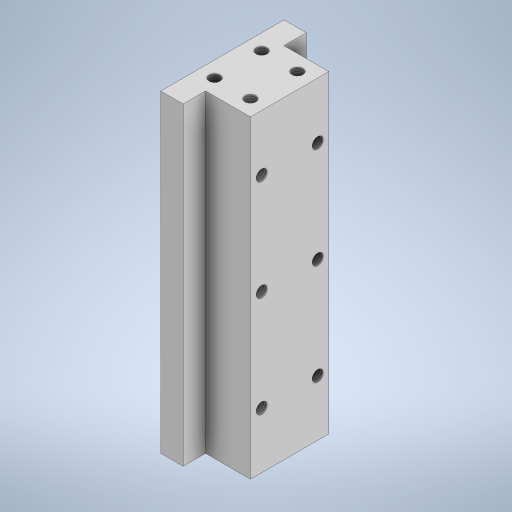
# Autodesk Inventor part: Fuhrung
Saved by Autodesk Inventor 2023 (Build 270158000, 158)
## iProperties
Created: 2023-05-10
Part Number: Fuhrung
Material: Generic
Document SubType Name: Modeling
Designer: dell
Density: 1 g/cm^3
Appearance: Default
Author: dell
Autodesk Inventor part; units mm, degrees
ref_plane "YZ Plane" through (0, 0, 0) normal (1, 0, 0) x (0, 1, 0)
ref_plane "XZ Plane" through (0, 0, 0) normal (0, 1, 0) x (-1, 0, 0)
ref_plane "XY Plane" through (0, 0, 0) normal (0, 0, 1) x (1, 0, 0)
sketch "Sketch1" plane through (0, 0, 0) normal (0, 1, 0) x (-1, 0, 0)
  line L0 (-10, 17.5) -> (10, 17.5)
  line L1 (10, 17.5) -> (10, -17.5)
  line L2 (10, -17.5) -> (-10, -17.5)
  line L3 (-10, -17.5) -> (-10, 17.5)
  line L4 (-10, 17.5) -> (10, -17.5) construction
  line L5 (10, 17.5) -> (-10, -17.5) construction
  point P0 (0, 0)
  dimension "d0" = 35
  dimension "d1" = 20
  constraints: 12 end point, 2 midpoint, 2 parallel, 1 horizontal, 1 perpendicular
  measures "d0" distance of L0.end L1.end
  measures "d1" distance of L1.end L2.end
extrude "Extrusion1" add sketch "Sketch1" along normal blind 140
sketch "Sketch2" plane through (0, 140, 0) normal (0, 1, 0) x (1, 0, 0)
  line L0 (-10, 27.5) -> (-10, -27.5)
  line L1 (-10, -27.5) -> (-20, -27.5)
  line L2 (-10, 27.5) -> (-20, 27.5)
  line L3 (-20, 27.5) -> (-20, -27.5)
  line L4 (-10, 17.5) -> (-10, -17.5) projected
  point P0 (0, 0)
  dimension "d4" = 55
  dimension "d5" = 0
  dimension "d6" = 10
  dimension "d7" = 27.5
  constraints: 8 end point, 2 horizontal, 2 vertical
  measures "d4" distance of L2.end L1.end
  measures "d5" distance between parallel lines of L0 L4
  measures "d6" distance between parallel lines of L0 L3
  measures "d7" distance from line of point (0, 0) L2
extrude "Extrusion2" add sketch "Sketch2" against normal blind 140
sketch "Sketch3" plane through (0, 140, 0) normal (0, 1, 0) x (1, 0, 0)
  line L0 (10, -17.5) -> (10, 17.5) projected
  point P0 (0, 0)
  point P1 (3, -10.5)
  dimension "d10" = 7
  dimension "d11" = 10.5
  measures "d10" distance from line of L0 point (3, -10.5)
  measures "d11" vertical distance of point (3, -10.5) point (0, 0)
hole "Hole1" at (3, 140, 10.5) direction (0, -1, 0) diameter 4.917 depth 20 tip angle 118 thread size "M6x1" class "6H" standard "ISO Metric profile"
pattern_linear "Rectangular Pattern1" count 2 spacing 16 along (-1, 0, 0) count 2 spacing 21 along (0, 0, -1) of "Hole1"
sketch "Sketch4" plane through (0, 0, 0) normal (0, -1, 0) x (1, 0, 0)
  line L0 (10, 17.5) -> (10, -17.5) projected
  point P0 (0, 0)
  point P1 (-13, -10.5)
  point P2 (-13, 10.5)
  point P3 (2, 0)
  dimension "d25" = 21
  dimension "d27" = 10.5
  dimension "d28" = 23
  dimension "d29" = 23
  dimension "d30" = 8
  dimension "d31" = 15
  measures "d25" distance of point (-13, -10.5) point (-13, 10.5)
  measures "d27" vertical distance of point (0, 0) point (-13, -10.5)
  measures "d28" distance from line of L0 point (-13, -10.5)
  measures "d29" distance from line of L0 point (-13, 10.5)
  measures "d30" distance from line of L0 point (2, 0)
  measures "d31" horizontal distance of point (-13, 10.5) point (2, 0)
hole "Hole2" at (-13, 0, -10.5) at (-13, 0, 10.5) at (2, 0, 0) direction (0, 1, 0) diameter 6.647 depth 20 tip angle 118 thread size "M8x1.25" class "6H" standard "ISO Metric profile"
sketch "Sketch5" plane through (10, 0, 17.5) normal (1, 0, 0) x (0, 0, -1)
  line L0 (0, 0) -> (35, 0) projected
  point P0 (17.5, 0)
  point P1 (30, 25)
  point P2 (17.5, 0)
  point P3 (17.5, 0)
  dimension "d39" = 25
  dimension "d40" = 12.5
  constraints: 2 midpoint
  measures "d39" vertical distance of point (17.5, 0) point (30, 25)
  measures "d40" horizontal distance of point (17.5, 0) point (30, 25)
hole "Hole3" at (10, 25, -12.5) direction (-1, 0, 0) diameter 4.917 depth 15 tip angle 118 thread size "M6x1" class "6H" standard "ISO Metric profile"
pattern_linear "Rectangular Pattern2" count 2 spacing 25 along (0, 0, 1) count 3 spacing 45 along (0, 1, 0) of "Hole3"
body "Solid1"
